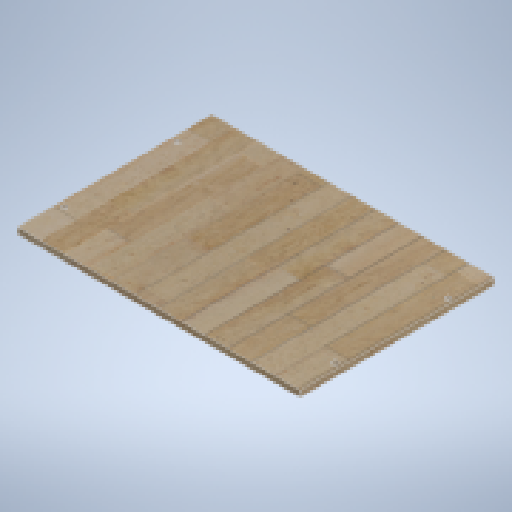
# Autodesk Inventor part: фанера1
Saved by Autodesk Inventor 2026.2 (Build 302298000, 298)
## iProperties
Created: 2026-05-20
Part Number: фанера1
Material: Wood (Maple)
Document SubType Name: Sheet Metal
Designer: admin
Density: 0.67 g/cm^3
Sheet Metal Rule: Default_mm
Appearance: Natural Maple - Glossy Dark Tint
Author: admin
Autodesk Inventor part; units mm, degrees
ref_plane "YZ Plane" through (0, 0, 0) normal (1, 0, 0) x (0, 1, 0)
ref_plane "XZ Plane" through (0, 0, 0) normal (0, 1, 0) x (-1, 0, 0)
ref_plane "XY Plane" through (0, 0, 0) normal (0, 0, 1) x (1, 0, 0)
sketch "Sketch1" plane through (0, 0, 0) normal (0, 1, 0) x (-1, 0, 0)
  line L0 (345, -237.5) -> (-345, -237.5)
  line L1 (-345, -237.5) -> (-345, 237.5)
  line L2 (-345, 237.5) -> (345, 237.5)
  line L3 (345, 237.5) -> (345, -237.5)
  line L4 (345, -237.5) -> (-345, 237.5) construction
  line L5 (-345, -237.5) -> (345, 237.5) construction
  point P0 (0, 0)
  dimension "d0" = 690
  dimension "d1" = 475
  measures "d0" distance of L1.end L2.end
  measures "d1" distance of L0.end L1.end
extrude "Plate1" add sketch "Sketch1" along normal blind 15
sketch "Sketch2" plane through (0, 15, 0) normal (0, 1, 0) x (1, 0, 0)
  line L0 (-345, -237.5) -> (-345, 237.5) construction
  line L1 (345, -237.5) -> (-345, -237.5) construction
  line L2 (345, 237.5) -> (345, -237.5) construction
  line L3 (-345, 237.5) -> (345, 237.5) construction
  line L4 (330, -237.5) -> (330, 237.5) construction
  line L5 (345, 0) -> (0, 0) construction
  point P0 (330, -137.5)
  point P1 (330, 137.5)
  dimension "d4" = 330
  dimension "d5" = 275
  dimension "d6" = 100
  dimension "d7" = 100
  constraints: 4 end point, 4 point on line, 1 horizontal, 1 midpoint, 1 perpendicular, 1 symmetric about line
  measures "d4" distance from line of L5.end L4
  measures "d5" distance of point (330, 137.5) point (330, -137.5)
  measures "d6" distance from line of L3 point (330, 137.5)
  measures "d7" distance from line of L1 point (330, -137.5)
hole "Hole1" at (330, 15, 137.5) at (330, 15, -137.5) direction (0, -1, 0) diameter 10 end through all counterbore diameter 14 counterbore depth 5
mirror "Mirror1" about plane through (0, 0, 0) normal (1, 0, 0) of "Hole1"
equation "\"d13\" = Thickness"
equation "\"d2\" = Thickness"
equation "\"BendRadius\" = Thickness"
equation "\"BendReliefWidth\" = Thickness"
equation "\"BendReliefDepth\" = 0.5 * Thickness"
equation "\"TransitionRadius\" = BendRadius"
equation "\"JacobiRadiusSize\" = BendRadius"
equation "\"GapSize\" = Thickness"
equation "\"Thickness\" = 15"
body "Solid1"
